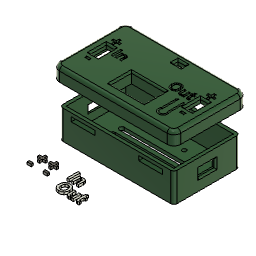
Buck Converter case v16 (Autodesk Fusion 360 design; units mm, degrees)
Autodesk Fusion 360 part; units mm, degrees
sketch "Box Main Sketch" plane through (0, 0, 0) normal (0, 0, 1) x (1, 0, 0)
  line L0 (0.0536, 74.9656) -> (0.0536, -63.0356) construction
  line L1 (-90.0982, 0.0562) -> (119.6914, 0.0562) construction
  line L2 (-33.4464, 18.5562) -> (33.5536, 18.5562)
  line L3 (33.5536, 18.5562) -> (33.5536, -18.4438)
  line L4 (33.5536, -18.4438) -> (-33.4464, -18.4438)
  line L5 (-33.4464, -18.4438) -> (-33.4464, 18.5562)
  line L6 (-35.4464, -18.4438) -> (-35.4464, 18.5562)
  line L7 (-33.4464, 20.5562) -> (33.5536, 20.5562)
  line L8 (35.5536, 18.5562) -> (35.5536, -18.4438)
  line L9 (33.5536, -20.4438) -> (-33.4464, -20.4438)
  arc A0 (35.5536, 18.5562) -> (33.5536, 20.5562) centre (33.5536, 18.5562) ccw
  arc A1 (33.5536, -20.4438) -> (35.5536, -18.4438) centre (33.5536, -18.4438) ccw
  arc A2 (-35.4464, -18.4438) -> (-33.4464, -20.4438) centre (-33.4464, -18.4438) ccw
  line L10 (-30.4464, 24.003) -> (-30.4464, 15.5562) construction
  circle A3 centre (-30.4464, 15.5562) radius 1.4
  circle A4 centre (30.5536, 15.5562) radius 1.4
  circle A5 centre (-30.4464, -15.4438) radius 1.4
  circle A6 centre (30.5536, -15.4438) radius 1.4
  line L11 (-33.4464, -18.4438) -> (-25.4464, -18.4438) construction
  line L12 (33.5536, 18.5562) -> (25.5536, 18.5562) construction
  line L13 (33.5536, 18.5562) -> (33.5536, 10.5562)
  arc A7 (-27.4464, -15.4438) -> (-25.4464, -18.4438) centre (-24.6377, -15.738) ccw
  arc A8 (-33.4464, -10.4438) -> (-30.4464, -12.4438) centre (-30.4464, -9.1938) ccw
  arc A9 (-25.4464, 18.5562) -> (-27.4464, 15.5562) centre (-24.1964, 15.5562) ccw
  arc A10 (-30.4464, 12.5562) -> (-33.4464, 10.5562) centre (-30.4464, 9.3062) ccw
  arc A11 (27.5536, 15.5562) -> (25.5536, 18.5562) centre (24.3036, 15.5562) ccw
  arc A12 (33.5536, 10.5562) -> (30.5536, 12.5562) centre (31.0441, 10.0418) ccw
  arc A13 (30.5479, -12.4438) -> (33.5536, -10.4438) centre (30.955, -9.7971) ccw
  arc A14 (25.5536, -18.4438) -> (27.5536, -15.4438) centre (24.3036, -15.4438) ccw
  arc A15 (-27.4617, -15.7469) -> (-30.4464, -12.4438) centre (-30.4464, -15.4438) ccw
  arc A16 (30.9836, -12.4748) -> (27.5536, -15.4438) centre (30.5536, -15.4438) ccw
  arc A17 (27.5536, 15.5562) -> (31.0831, 12.6033) centre (30.5536, 15.5562) ccw
  arc A18 (-30.4464, 12.5562) -> (-27.4464, 15.5562) centre (-30.4464, 15.5562) ccw
  line L14 (-20.0548, 1.2518) -> (20.324, 1.2485)
  arc A19 (20.324, 1.2485) -> (20.3242, 4.2485) centre (20.3241, 2.7485) ccw
  line L15 (20.3242, 4.2485) -> (-20.0545, 4.2518)
  arc A20 (-20.0545, 4.2518) -> (-20.0548, 1.2518) centre (-20.0547, 2.7518) ccw
  line L16 (-20.0547, -4.2975) -> (20.3241, -4.2975)
  arc A21 (20.3241, -4.2975) -> (20.3241, -1.2975) centre (20.3241, -2.7975) ccw
  line L17 (20.3241, -1.2975) -> (-20.0547, -1.2975)
  arc A22 (-20.0547, -1.2975) -> (-20.0547, -4.2975) centre (-20.0547, -2.7975) ccw
  line L18 (-20.0547, -2.7975) -> (20.3241, -2.7975) construction
  line L19 (-20.0547, 0.0562) -> (20.0734, 0.0562) construction
  line L20 (-20.0547, -9.6836) -> (20.3241, -9.6836)
  arc A23 (20.3241, -9.6836) -> (20.3241, -6.6836) centre (20.3241, -8.1836) ccw
  line L21 (20.3241, -6.6836) -> (-20.0547, -6.6836)
  arc A24 (-20.0547, -6.6836) -> (-20.0547, -9.6836) centre (-20.0547, -8.1836) ccw
  line L22 (-20.0547, -8.1836) -> (20.3241, -8.1836) construction
  line L23 (-20.0547, -15.4896) -> (20.3241, -15.4896)
  arc A25 (20.3241, -15.4896) -> (20.3241, -12.4896) centre (20.3241, -13.9896) ccw
  line L24 (20.3241, -12.4896) -> (-20.0547, -12.4896)
  arc A26 (-20.0547, -12.4896) -> (-20.0547, -15.4896) centre (-20.0547, -13.9896) ccw
  line L25 (-20.0547, -13.9896) -> (20.3241, -13.9896) construction
  arc A27 (-33.4464, 20.5562) -> (-35.4464, 18.5562) centre (-33.4464, 18.5562) ccw
  line L26 (-33.4464, 5.5562) -> (-35.4464, 5.5562)
  line L27 (35.5536, 5.5562) -> (33.5536, 5.5562)
  line L28 (35.5536, 7.5562) -> (33.5536, 7.5562) construction
  line L29 (-33.4464, 7.5562) -> (-35.4464, 7.5562) construction
  circle A28 centre (-29.0547, 10.5065) radius 1.25
  line L30 (-29.0547, 10.5065) -> (22.3046, 10.5554) construction
  line L31 (-14.904, 20.5562) -> (-14.904, 11.5562) construction
  circle A29 centre (11.0453, 10.5447) radius 1.25
  line L32 (-29.0547, 10.5065) -> (-29.0547, 26.528) construction
  line L33 (11.0453, 10.5447) -> (11.0453, 25.7111) construction
  line L34 (-29.0547, 24.003) -> (11.0453, 24.003) construction
  point P0 (30.5536, -15.4438)
  dimension "d1" = 67
  dimension "d2" = 37
  dimension "d4" = 2
  dimension "d9" = 2.8
  dimension "d65" = 3
  dimension "d66" = 3
  dimension "d68" = 3
  dimension "d69" = 3
  dimension "d80" = 2
  dimension "d82" = 2
  dimension "d83" = 2
  dimension "d181" = 2.5
  dimension "d194" = 9
  dimension "d195" = 2.5
  dimension "d206" = 40.1
  constraint vertical L0
  constraint perpendicular L0 L1
  constraint horizontal L2
  constraint vertical L3
  constraint horizontal L4
  constraint vertical L5
  constraint symmetric L0 L3 L5
  constraint symmetric L1 L2 L4
  constraint tangent L7 A0
  constraint tangent L8 A0
  constraint tangent L8 A1
  constraint tangent L9 A1
  constraint equal A0 A1
  constraint tangent L6 A2
  constraint tangent L9 A2
  constraint equal A0 A2
  constraint coincident L10.end A3.centre
  constraint coincident L4.end L5.start
  constraint coincident L4 L11.end
  constraint coincident L2.end L3.start
  constraint perpendicular L2 L13
  constraint coincident A7.start A15
  constraint tangent A8 A15
  constraint coincident L5 A8.start
  constraint tangent A9 A18
  constraint coincident L2 A9.start
  constraint tangent A10 A18
  constraint coincident L5 A10.end
  constraint tangent A11 A17
  constraint coincident A12.end A17
  constraint coincident L3 A13.end
  constraint coincident A13.start A16
  constraint tangent A14 A16
  constraint coincident L4 A14.start
  constraint coincident A7 A15.start
  constraint concentric A6 A16
  constraint coincident A13 A16.start
  constraint coincident A12 A17.end
  constraint tangent L14 A19
  constraint tangent A19 L15
  constraint parallel L14 L15
  constraint tangent L15 A20
  constraint tangent L14 A20
  constraint tangent L16 A21
  constraint tangent A21 L17
  constraint parallel L16 L17
  constraint tangent L17 A22
  constraint tangent L16 A22
  constraint coincident L1 L19.start
  constraint tangent L20 A23
  constraint tangent A23 L21
  constraint parallel L20 L21
  constraint tangent L21 A24
  constraint tangent L20 A24
  constraint tangent L23 A25
  constraint tangent A25 L24
  constraint parallel L23 L24
  constraint tangent L24 A26
  constraint tangent L23 A26
  constraint tangent L6 A27
  constraint tangent L7 A27
  constraint coincident L5 L26.start
  constraint coincident L6 L26.end
  constraint perpendicular L6 L26
  constraint coincident L8 L27.start
  constraint coincident L3 L27.end
  constraint coincident L7 L31.start
  constraint perpendicular L2 L31
  constraint coincident L30 A29.centre
  constraint coincident A28.centre L30.start
  constraint perpendicular L2 L32
  constraint coincident A29.centre L33.start
  constraint perpendicular L7 L33
  constraint coincident L32 L34.start
  constraint coincident L33 L34.end
  constraint perpendicular L33 L34
  measures "d1" distance of L2.start L2.end
  measures "d2" distance of L2.start L4.end
  measures "d4" radius of A0
  measures "d9" diameter of A3
  measures "d65" diameter of A19
  measures "d66" diameter of A21
  measures "d68" diameter of A23
  measures "d69" diameter of A25
  measures "d80" radius of A27
  measures "d82" distance of L27
  measures "d83" distance of L26
  measures "d181" diameter of A28
  measures "d194" distance of L31.start L31.end
  measures "d195" diameter of A29
  measures "d206" distance of L34.start L34.end
extrude "Bottom of Box" add sketch "Box Main Sketch" along normal blind 2 contours L2 L3 L4 L5 A7 A8 A9 A10 A11 A12 A13 A14 A15 A16 A17 A18 | L14 A19 L15 A20 | L16 A21 L17 A22 | L20 A23 L21 A24 | L23 A25 L24 A26 | A28 | A29 makes body 1
extrude "Bottom Corners" add sketch "Box Main Sketch" along normal blind 5 contours L2 L5 A9 A10 A18 | L2 L3 L13 A11 A12 A17 | L4 L5 A7 A8 A15 | L3 L4 A13 A14 A16 | A3 | A4 | A5 | A6 bodies 1
extrude "Main Box Body" add sketch "Box Main Sketch" along normal blind 18 contours L2 L3 L5 L6 L7 L8 A0 L13 A27 L26 L27 | L3 L4 L5 L6 L8 L9 A1 A2 L26 L27 bodies 1
sketch "End of Box for input" plane through (33.5536, 0, 0) normal (-1, 0, 0) x (0, -1, 0)
  line L0 (10.4438, 5) -> (18.4438, 5)
  line L1 (18.4438, 5) -> (18.4438, 18)
  line L2 (18.4438, 18) -> (-18.5562, 18)
  line L3 (-18.5562, 18) -> (-18.5562, 5)
  line L4 (-18.5562, 5) -> (-10.5562, 5)
  line L5 (-10.5562, 5) -> (-10.5562, 2)
  line L6 (-10.5562, 2) -> (10.4438, 2)
  line L7 (10.4438, 2) -> (10.4438, 5)
  line L8 (4.6555, 6.9963) -> (-5.3445, 6.9963)
  line L9 (-5.3445, 6.9963) -> (-5.3445, 11.9963)
  line L10 (-5.3445, 11.9963) -> (4.6555, 11.9963)
  line L11 (4.6555, 11.9963) -> (4.6555, 6.9963)
  line L12 (0, 0) -> (0, 7) construction
  dimension "d54" = 10
  dimension "d55" = 5
  dimension "d72" = 7
  constraint horizontal L8
  constraint vertical L9
  constraint horizontal L10
  constraint vertical L11
  constraint coincident L12.start origin
  constraint perpendicular L0 L12
  measures "d54" distance of L8.start L8.end
  measures "d55" distance of L8.start L10.end
  measures "d72" distance of L12.start L12.end
extrude "End Wire Holes" cut sketch "End of Box for input" against normal blind 2 contours L8 L9 L10 L11 bodies 1
sketch "End of box for output" plane through (-35.4464, 0, 0) normal (-1, 0, 0) x (0, -1, 0)
  line L0 (-18.5562, 0) -> (18.4438, 0)
  line L1 (18.4438, 0) -> (18.4438, 18)
  line L2 (18.4438, 18) -> (-18.5562, 18)
  line L3 (-5.1039, 6.9396) -> (4.8961, 6.9396)
  line L4 (4.8961, 6.9396) -> (4.8961, 11.9396)
  line L5 (4.8961, 11.9396) -> (-5.1039, 11.9396)
  line L6 (-5.1039, 11.9396) -> (-5.1039, 6.9396)
  line L7 (3.7468, 0) -> (3.7468, 7) construction
  line L8 (-18.5562, 18) -> (-18.5562, 0)
  dimension "d43" = 10
  dimension "d44" = 5
  dimension "d58" = 7
  constraint horizontal L3
  constraint vertical L4
  constraint horizontal L5
  constraint vertical L6
  constraint coincident L0 L7.start
  constraint perpendicular L3 L7
  measures "d43" distance of L3.start L3.end
  measures "d44" distance of L3.start L5.end
  measures "d58" distance of L7.start L7.end
extrude "End Wire Hole" cut sketch "End of box for output" against normal blind 2 contours L3 L4 L5 L6 bodies 1
fillet "wire Hole" radius 1 4 edges at (-35.4464, 0.1039, 11.9396) (-35.4464, 5.1039, 9.4396) (-35.4464, 0.1039, 6.9396) (-35.4464, -4.8961, 9.4396) on bodies 1
fillet "Wire Hole" radius 1 4 edges at (35.5536, 0.3445, 6.9963) (35.5536, 5.3445, 9.4963) (35.5536, 0.3445, 11.9963) (35.5536, -4.6555, 9.4963) on bodies 1
extrude "Mounting Posts" add sketch "Box Main Sketch" along normal blind 8 contours A3 | A4 | A5 | A6 bodies 1
extrude "Vent Holes in bottom" cut sketch "Box Main Sketch" along normal blind 2 contours L14 A19 L15 A20 | L16 A21 L17 A22 | L20 A23 L21 A24 | L23 A25 L24 A26 bodies 1
sketch "Box Catch holes" plane through (0, 20.5562, 0) normal (0, 1, 0) x (-1, 0, 0)
  line L0 (-33.5536, 0) -> (33.4464, 0)
  line L1 (33.4464, 0) -> (33.4464, 18)
  line L2 (33.4464, 18) -> (-33.5536, 18)
  line L3 (-33.5536, 18) -> (-33.5536, 0)
  line L4 (33.4464, 16.015) -> (28.4464, 16.015) construction
  line L5 (28.4464, 16.015) -> (13.4464, 16.015)
  line L6 (13.4464, 16.015) -> (13.4464, 13.015)
  line L7 (13.4464, 13.015) -> (28.4464, 13.015)
  line L8 (28.4464, 13.015) -> (28.4464, 16.015)
  line L9 (-28.5536, 13.0366) -> (-13.5536, 13.0366)
  line L10 (-28.5536, 16.0366) -> (-28.5536, 13.0366)
  line L11 (-13.5536, 16.0366) -> (-28.5536, 16.0366)
  line L12 (-13.5536, 13.0366) -> (-13.5536, 16.0366)
  dimension "d85" = 5
  dimension "d87" = 15
  dimension "d88" = 3
  dimension "d89" = 15
  dimension "d90" = 3
  constraint coincident L1 L4.start
  constraint perpendicular L1 L4
  constraint horizontal L5
  constraint vertical L6
  constraint horizontal L7
  constraint vertical L8
  constraint horizontal L11
  constraint vertical L10
  constraint horizontal L9
  constraint vertical L12
  measures "d85" distance of L4.start L4.end
  measures "d87" distance of L4.end L5.end
  measures "d88" distance of L4.end L7.end
  measures "d89" distance of L10.start L11.start
  measures "d90" distance of L9.end L11.start
extrude "Back Catch Slots" cut sketch "Box Catch holes" against normal blind 1.5 draft -45 contours L5 L6 L7 L8 | L9 L10 L11 L12 bodies 1
mirror "Front Catches" about plane through (0, 0, 0) normal (0, 1, 0) of "Back Catch Slots"
sketch "Lid Rim" plane through (0, 0, 18) normal (0, 0, 1) x (-1, 0, 0) in component "Lid"
  line L0 (33.4464, -18.5562) -> (-33.5536, -18.5562)
  line L1 (-33.5536, -18.5562) -> (-33.5536, 18.4438)
  line L2 (-33.5536, 18.4438) -> (33.4464, 18.4438)
  line L3 (33.4464, 18.4438) -> (33.4464, -18.5562)
  arc A0 (-35.5536, -18.5562) -> (-33.5536, -20.5562) centre (-33.5536, -18.5562) ccw
  line L4 (-33.5536, -20.5562) -> (33.4464, -20.5562)
  arc A1 (33.4464, -20.5562) -> (35.4464, -18.5562) centre (33.4464, -18.5562) ccw
  line L5 (35.4464, -18.5562) -> (35.4464, 18.4438)
  arc A2 (35.4464, 18.4438) -> (33.4464, 20.4438) centre (33.4464, 18.4438) ccw
  line L6 (33.4464, 20.4438) -> (-33.5536, 20.4438)
  arc A3 (-33.5536, 20.4438) -> (-35.5536, 18.4438) centre (-33.5536, 18.4438) ccw
  line L7 (-35.5536, 18.4438) -> (-35.5536, -18.5562)
  line L8 (-33.5536, 20.4438) -> (33.4464, 20.4438)
  arc A4 (-33.5536, 20.4438) -> (-35.5536, 18.4438) centre (-33.5536, 18.4438) ccw
  line L9 (-35.5536, -18.5562) -> (-35.5536, 18.4438)
  arc A5 (-35.5536, -18.5562) -> (-33.5536, -20.5562) centre (-33.5536, -18.5562) ccw
  line L10 (33.4464, -20.5562) -> (-33.5536, -20.5562)
  arc A6 (33.4464, -20.5562) -> (35.4464, -18.5562) centre (33.4464, -18.5562) ccw
  line L11 (35.4464, 18.4438) -> (35.4464, -18.5562)
  arc A7 (35.4464, 18.4438) -> (33.4464, 20.4438) centre (33.4464, 18.4438) ccw
  line L12 (-37.7536, 18.4438) -> (-37.7536, -18.5562)
  arc A8 (-37.7536, -18.5562) -> (-33.5536, -22.7562) centre (-33.5536, -18.5562) ccw
  line L13 (-33.5536, -22.7562) -> (33.4464, -22.7562)
  arc A9 (33.4464, -22.7562) -> (37.6464, -18.5562) centre (33.4464, -18.5562) ccw
  line L14 (37.6464, -18.5562) -> (37.6464, 18.4438)
  arc A10 (37.6464, 18.4438) -> (33.4464, 22.6438) centre (33.4464, 18.4438) ccw
  line L15 (33.4464, 22.6438) -> (-33.5536, 22.6438)
  arc A11 (-33.5536, 22.6438) -> (-37.7536, 18.4438) centre (-33.5536, 18.4438) ccw
  line L16 (-35.7536, 18.4438) -> (-35.7536, -18.5562)
  arc A12 (-35.7536, -18.5562) -> (-33.5536, -20.7562) centre (-33.5536, -18.5562) ccw
  line L17 (-33.5536, -20.7562) -> (33.4464, -20.7562)
  arc A13 (33.4464, -20.7562) -> (35.6464, -18.5562) centre (33.4464, -18.5562) ccw
  line L18 (35.6464, -18.5562) -> (35.6464, 18.4438)
  arc A14 (35.6464, 18.4438) -> (33.4464, 20.6438) centre (33.4464, 18.4438) ccw
  line L19 (33.4464, 20.6438) -> (-33.5536, 20.6438)
  arc A15 (-33.5536, 20.6438) -> (-35.7536, 18.4438) centre (-33.5536, 18.4438) ccw
  constraint concentric A0 A8
  constraint concentric A1 A9
  constraint concentric A2 A10
  constraint concentric A3 A11
  constraint tangent L15 A11
  constraint tangent L14 A10
  constraint tangent A9 L14
  constraint tangent L13 A9
  constraint tangent A8 L13
  constraint tangent A10 L15
  constraint tangent L12 A8
  constraint tangent L12 A11
  constraint concentric A0 A12
  constraint concentric A1 A13
  constraint concentric A2 A14
  constraint concentric A3 A15
  constraint tangent A14 L19
  constraint tangent L18 A14
  constraint tangent L19 A15
  constraint tangent A13 L18
  constraint tangent L16 A15
  constraint tangent L17 A13
  constraint tangent A12 L17
  constraint tangent L16 A12
extrude "Lid Main Part" add sketch "Lid Rim" against normal blind 5 separate body contours L12 A8 L13 A9 L14 A10 L15 A11 makes body 2 in component "Lid"
sketch "Lid top" plane through (0, 0, 18) normal (0, 0, 1) x (1, 0, 0) in component "Lid"
  line L0 (33.5536, 22.7562) -> (-33.4464, 22.7562)
  arc A0 (37.7536, 18.5562) -> (33.5536, 22.7562) centre (33.5536, 18.5562) ccw
  line L1 (37.7536, -18.4438) -> (37.7536, 18.5562)
  arc A1 (33.5536, -22.6438) -> (37.7536, -18.4438) centre (33.5536, -18.4438) ccw
  line L2 (-33.4464, -22.6438) -> (33.5536, -22.6438)
  arc A2 (-37.6464, -18.4438) -> (-33.4464, -22.6438) centre (-33.4464, -18.4438) ccw
  line L3 (-37.6464, 18.5562) -> (-37.6464, -18.4438)
  arc A3 (-33.4464, 22.7562) -> (-37.6464, 18.5562) centre (-33.4464, 18.5562) ccw
  line L4 (31.7125, -5.0985) -> (26.7125, -5.0985)
  line L5 (26.7125, -5.0985) -> (26.7125, 4.9015)
  line L6 (26.7125, 4.9015) -> (31.7125, 4.9015)
  line L7 (31.7125, 4.9015) -> (31.7125, -5.0985)
  line L8 (-37.6464, 2.2618) -> (-33.6464, 2.2618) construction
  line L9 (-26.7875, 4.9015) -> (-26.7875, -5.0985)
  line L10 (-26.7875, -5.0985) -> (-31.7875, -5.0985)
  line L11 (-31.7875, -5.0985) -> (-31.7875, 4.9015)
  line L12 (-31.7875, 4.9015) -> (-26.7875, 4.9015)
  line L13 (-0.6158, 18.2562) -> (4.3842, 18.2562)
  line L14 (4.3842, 18.2562) -> (4.3842, 15.2562)
  line L15 (4.3842, 15.2562) -> (-0.6158, 15.2562)
  line L16 (-0.6158, 15.2562) -> (-0.6158, 18.2562)
  line L17 (-35.4464, 18.5562) -> (-35.4464, -18.4438)
  line L18 (33.5536, 20.5562) -> (-33.4464, 20.5562)
  line L19 (35.5536, -18.4438) -> (35.5536, 18.5562)
  line L20 (-33.4464, -20.4438) -> (33.5536, -20.4438)
  line L21 (-35.4464, -18.4438) -> (-35.4464, 18.5562)
  line L22 (-33.4464, 20.5562) -> (33.5536, 20.5562)
  line L23 (33.5536, -20.4438) -> (-33.4464, -20.4438)
  line L24 (35.5536, 18.5562) -> (35.5536, -18.4438)
  line L25 (-8.8611, -20.4438) -> (-8.8611, -15.4438) construction
  line L26 (-8.8611, -15.4438) -> (12.1389, -15.4438)
  line L27 (12.1389, -15.4438) -> (12.1389, -2.4438)
  line L28 (12.1389, -2.4438) -> (-8.8611, -2.4438)
  line L29 (-8.8611, -2.4438) -> (-8.8611, -15.4438)
  line L30 (-10.3611, -0.9438) -> (-10.3611, -16.9438)
  line L31 (-10.3611, -16.9438) -> (13.6389, -16.9438)
  line L32 (13.6389, -16.9438) -> (13.6389, -0.9438)
  line L33 (13.6389, -0.9438) -> (-10.3611, -0.9438)
  line L34 (22.4453, -20.4438) -> (22.4453, -13.9438) construction
  line L35 (24.0234, -12.7383) -> (24.0234, -2.5519)
  line L36 (24.0234, -2.5519) -> (20.8495, -2.5519)
  line L37 (20.8495, -2.5519) -> (20.8495, -12.7383)
  line L38 (25.0234, -12.4097) -> (25.0234, -3.5519)
  line L39 (19.8495, -3.5519) -> (19.8495, -12.4399)
  arc A4 (19.8495, -12.4399) -> (25.0234, -12.4097) centre (22.4453, -13.9438) ccw
  arc A5 (20.8495, -12.7383) -> (24.0234, -12.7152) centre (22.4453, -13.9438) ccw
  line L40 (20.8495, -2.5519) -> (19.7948, -3.6066)
  line L41 (20.8495, -2.5519) -> (22.3411, -2.5519) construction
  line L42 (24.0234, -2.5519) -> (24.9601, -3.4885)
  line L43 (25.0234, -2.5519) -> (25.348, -2.5519) construction
  line L44 (24.9601, -3.4885) -> (25.0234, -3.5519)
  circle A6 centre (22.4453, -13.9438) radius 1.875
  dimension "d113" = 5
  dimension "d114" = 10
  dimension "d116" = 4
  dimension "d117" = 5
  dimension "d118" = 10
  dimension "d121" = 5
  dimension "d122" = 3
  dimension "d126" = 5
  dimension "d127" = 21
  dimension "d128" = 13
  dimension "d129" = 1.5
  dimension "d143" = 6.5
  dimension "d144" = 4
  dimension "d147" = 135
  dimension "d148" = 45
  dimension "d149" = 3.75
  constraint horizontal L4
  constraint vertical L5
  constraint horizontal L6
  constraint vertical L7
  constraint coincident L3 L8.start
  constraint perpendicular L3 L8
  constraint horizontal L10
  constraint vertical L11
  constraint horizontal L12
  constraint vertical L9
  constraint horizontal L13
  constraint vertical L14
  constraint horizontal L15
  constraint vertical L16
  constraint coincident L20 L25.start
  constraint perpendicular L20 L25
  constraint horizontal L26
  constraint vertical L27
  constraint horizontal L28
  constraint vertical L29
  constraint coincident L23 L34.start
  constraint perpendicular L23 L34
  constraint coincident L34.end A4.centre
  constraint vertical L35
  constraint horizontal L36
  constraint vertical L37
  constraint concentric A4 A5
  constraint coincident L35 A5.end
  constraint horizontal L41
  constraint coincident L40 L39.start
  constraint horizontal L43
  constraint parallel L42 L44
  constraint concentric A4 A6
  measures "d113" distance of L4.start L4.end
  measures "d114" distance of L4.start L6.end
  measures "d116" distance of L8.start L8.end
  measures "d117" distance of L9.end L10.end
  measures "d118" distance of L9.end L9.start
  measures "d121" distance of L13.start L13.end
  measures "d122" distance of L13.start L15.end
  measures "d126" distance of L25.start L25.end
  measures "d127" distance of L25.end L26.end
  measures "d128" distance of L25.end L28.end
  measures "d143" distance of L34.start L34.end
  measures "d144" diameter of A5
  measures "d147" angle of L40 L41
  measures "d148" angle of L42 L43
  measures "d149" diameter of A6
extrude "Lid top (1)" add sketch "Lid top" along normal blind 3 contours L0 A0 L1 A1 L2 A2 L3 A3 | L4 L5 L6 L7 | L9 L10 L11 L12 | L13 L14 L15 L16 | L26 L27 L28 L29 | L30 L31 L32 L33 | L35 L36 L37 A5 | L35 L37 L38 L39 A4 A5 L40 L42 L44 | A6 bodies 2 in component "Lid"
fillet "Lid top (2)" radius 2 1 faces at (11.2203, -7.5105, 21) on bodies 2 in component "Lid"
sketch "Lid Catches" plane through (0, -20.6438, 0) normal (0, 1, 0) x (-1, 0, 0) in component "Lid"
  line L0 (33.4464, 18) -> (-33.5536, 18)
  line L1 (-33.5536, 18) -> (-33.5536, 13)
  line L2 (-33.5536, 13) -> (33.4464, 13)
  line L3 (33.4464, 13) -> (33.4464, 18)
  line L4 (-13.5536, 16.0366) -> (-13.5536, 13.0366)
  line L5 (-13.5536, 13.0366) -> (-28.5536, 13.0366)
  line L6 (-28.5536, 13.0366) -> (-28.5536, 16.0366)
  line L7 (13.4464, 13.015) -> (13.4464, 16.015)
  line L8 (28.4464, 13.015) -> (13.4464, 13.015)
  line L9 (28.4464, 16.015) -> (28.4464, 13.015)
  line L10 (-13.5536, 16.0366) -> (-28.5536, 16.0366)
  line L11 (-13.5536, 13.0366) -> (-13.5536, 16.0366)
  line L12 (-28.5536, 13.0366) -> (-13.5536, 13.0366)
  line L13 (-28.5536, 16.0366) -> (-28.5536, 13.0366)
  line L14 (13.4464, 16.015) -> (13.4464, 13.015)
  line L15 (13.4464, 13.015) -> (28.4464, 13.015)
  line L16 (28.4464, 13.015) -> (28.4464, 16.015)
  line L17 (28.4464, 16.015) -> (13.4464, 16.015)
extrude "Front Catch Pins" add sketch "Lid Catches" along normal blind 1.5 draft -45 contours L4 L5 L6 L10 L11 L12 L13 | L7 L8 L9 L14 L15 L16 L17 bodies 2 in component "Lid"
sketch "Other Lid Catches" plane through (0, 20.7562, 0) normal (0, -1, 0) x (1, 0, 0) in component "Lid"
  line L0 (33.5536, 18) -> (-33.4464, 18)
  line L1 (-33.4464, 18) -> (-33.4464, 13)
  line L2 (-33.4464, 13) -> (33.5536, 13)
  line L3 (33.5536, 13) -> (33.5536, 18)
  line L4 (28.4413, 15.9243) -> (28.4413, 13.149)
  line L5 (13.666, 15.9243) -> (28.4413, 15.9243)
  line L6 (13.666, 13.149) -> (13.666, 15.9243)
  line L7 (13.666, 15.9243) -> (28.4413, 15.9243)
  line L8 (28.4413, 15.9243) -> (28.4413, 13.149)
  line L9 (28.4413, 13.149) -> (13.666, 13.149)
  line L10 (13.666, 13.149) -> (13.666, 15.9243)
  line L11 (-28.334, 15.9026) -> (-13.5587, 15.9026)
  line L12 (-13.5587, 15.9026) -> (-13.5587, 13.1274)
  line L13 (-13.5587, 13.1274) -> (-28.334, 13.1274)
  line L14 (-28.334, 13.1274) -> (-28.334, 15.9026)
  line L15 (-33.4464, 0) -> (33.5536, 0)
  line L16 (33.5536, 0) -> (33.5536, 18)
  line L17 (33.5536, 18) -> (-33.4464, 18)
  line L18 (-33.4464, 18) -> (-33.4464, 0)
  line L19 (-13.5587, 15.9026) -> (-13.5587, 13.1274)
  line L20 (-28.334, 15.9026) -> (-13.5587, 15.9026)
  line L21 (-28.334, 13.1274) -> (-28.334, 15.9026)
  line L22 (-13.5587, 13.1274) -> (-28.334, 13.1274)
extrude "Rear Catch Pins" add sketch "Other Lid Catches" along normal blind 1.5 draft -45 contours L4 L5 L6 L7 L8 L9 L10 | L11 L12 L13 L14 L19 L20 L21 L22 bodies 2 in component "Lid"
extrude "Top Holes" cut sketch "Lid top" along normal blind 3 contours L4 L5 L6 L7 | L9 L10 L11 L12 | L13 L14 L15 L16 | L26 L27 L28 L29 | L35 L37 L38 L39 A4 A5 L40 L42 L44 bodies 2 in component "Lid"
extrude "Voltage Display hole" add sketch "Lid top" against normal blind 3.7 contours L30 L31 L32 L33 bodies 2 in component "Lid"
fillet "Screw Holes" radius 1 15 edges at (-26.7875, -0.0985, 21) (-29.2875, 4.9015, 21) (-31.7875, -0.0985, 21) (-29.2875, -5.0985, 21) (1.6389, -2.4438, 21) (-8.8611, -8.9438, 21) (1.6389, -15.4438, 21) (1.8842, 15.2562, 21) (26.7125, -0.0985, 21) (29.2125, -5.0985, 21) (31.7125, -0.0985, 21) (29.2125, 4.9015, 21) (4.3842, 16.7562, 21) (1.8842, 18.2562, 21) (-0.6158, 16.7562, 21) on bodies 2 in component "Lid"
fillet "Voltage Display" radius 1 1 edges at (12.1389, -8.9438, 21) on bodies 2 in component "Lid"
move_body "Move1" bodies 2 to x (1, 0, 0) y (0, 1, 0) z (0, 0, 1) at (0, 0, 35) in component "Lid"
move_body "Move2" bodies 2 to x (1, 0, 0) y (0, 1, 0) z (0, 0, 1) at (0, 0, -35) in component "Lid"
extrude "PushButton Pin" add sketch "Lid top" against normal blind 5.75 draft -3 contours A6 bodies 2 in component "Lid"
sketch "Emboss Letters" plane through (0, 0, 21) normal (0, 0, 1) x (-1, 0, 0) in component "Lid"
  arc A0 (33.4464, -20.7562) -> (35.6464, -18.5562) centre (33.4464, -18.5562) ccw
  line L0 (35.6464, -18.5562) -> (35.6464, 18.4438)
  arc A1 (35.6464, 18.4438) -> (33.4464, 20.6438) centre (33.4464, 18.4438) ccw
  line L1 (33.4464, 20.6438) -> (-33.5536, 20.6438)
  arc A2 (-33.5536, 20.6438) -> (-35.7536, 18.4438) centre (-33.5536, 18.4438) ccw
  line L2 (-35.7536, 18.4438) -> (-35.7536, -18.5562)
  arc A3 (-35.7536, -18.5562) -> (-33.5536, -20.7562) centre (-33.5536, -18.5562) ccw
  line L3 (-33.5536, -20.7562) -> (33.4464, -20.7562)
  line L4 (31.8884, -5.9664) -> (26.4793, -6.0573) construction
  line L5 (26.4793, -6.0573) -> (26.568, -11.3367) construction
  line L6 (26.568, -11.3367) -> (31.9771, -11.2458) construction
  line L7 (31.9771, -11.2458) -> (31.8884, -5.9664) construction
  line L8 (-27.1116, -5.9664) -> (-32.5207, -6.0573) construction
  line L9 (-32.5207, -6.0573) -> (-32.432, -11.3367) construction
  line L10 (-32.432, -11.3367) -> (-27.0229, -11.2458) construction
  line L11 (-27.0229, -11.2458) -> (-27.1116, -5.9664) construction
  line L12 (24.0133, 0.021) -> (14.3092, 0.0016) construction
  line L13 (14.3092, 0.0016) -> (14.3216, -6.2061) construction
  line L14 (14.3216, -6.2061) -> (24.0257, -6.1867) construction
  line L15 (24.0257, -6.1867) -> (24.0133, 0.021) construction
  line L16 (-10.495, 0.0928) -> (-24.7584, 0.1552) construction
  line L17 (-24.7584, 0.1552) -> (-24.7855, -6.0483) construction
  line L18 (-24.7855, -6.0483) -> (-10.5221, -6.1106) construction
  line L19 (-10.5221, -6.1106) -> (-10.495, 0.0928) construction
  line L20 (-13.1389, 16.4438) -> (9.8611, 16.4438)
  line L21 (9.8611, 16.4438) -> (9.8611, 1.4438)
  line L22 (9.8611, 1.4438) -> (-13.1389, 1.4438)
  line L23 (-13.1389, 1.4438) -> (-13.1389, 16.4438)
  line L24 (-5.3842, -19.2562) -> (-5.3842, -14.2562)
  line L25 (-5.3842, -14.2562) -> (1.6158, -14.2562)
  line L26 (1.6158, -14.2562) -> (1.6158, -19.2562)
  line L27 (1.6158, -19.2562) -> (-5.3842, -19.2562)
  line L28 (32.7875, -5.9015) -> (25.7875, -5.9015)
  line L29 (25.7875, -5.9015) -> (25.7875, 6.0985)
  line L30 (25.7875, 6.0985) -> (32.7875, 6.0985)
  line L31 (32.7875, 6.0985) -> (32.7875, -5.9015)
  line L32 (-20.8495, 2.5519) -> (-20.8495, 12.7383)
  arc A4 (-20.8495, 12.7383) -> (-24.0234, 12.7152) centre (-22.4453, 13.9438) ccw
  line L33 (-24.0234, 12.7152) -> (-24.0234, 2.5519)
  line L34 (-24.0234, 2.5519) -> (-25.0234, 3.5519)
  line L35 (-25.0234, 3.5519) -> (-25.0234, 12.4097)
  arc A5 (-19.8495, 12.4399) -> (-25.0234, 12.4097) centre (-22.4453, 13.9438) ccw
  line L36 (-19.8495, 12.4399) -> (-19.8495, 3.5519)
  line L37 (-19.8495, 3.5519) -> (-20.8495, 2.5519)
  line L38 (-32.7125, -5.9015) -> (-32.7125, 6.0985)
  line L39 (-32.7125, 6.0985) -> (-25.7125, 6.0985)
  line L40 (-25.7125, 6.0985) -> (-25.7125, -5.9015)
  line L41 (-25.7125, -5.9015) -> (-32.7125, -5.9015)
  line L42 (31.0051, 10.7007) -> (25.4979, 10.7007) construction
  line L43 (25.4979, 10.7007) -> (25.4979, 8.0454) construction
  line L44 (25.4979, 8.0454) -> (31.0051, 8.0454) construction
  line L45 (31.0051, 8.0454) -> (31.0051, 10.7007) construction
  line L46 (-27.9949, 10.7007) -> (-33.5021, 10.7007) construction
  line L47 (-33.5021, 10.7007) -> (-33.5021, 8.0454) construction
  line L48 (-33.5021, 8.0454) -> (-27.9949, 8.0454) construction
  line L49 (-27.9949, 8.0454) -> (-27.9949, 10.7007) construction
  dimension "d170" = 7
  dimension "d172" = 7
  dimension "d175" = 6
  dimension "d176" = 6
  dimension "d188" = 7
  dimension "d189" = 7
  text T0 "+" font "Arial" height 7 bold align left top in box 5.4099 x 5.2802 at (31.8884, -5.9664) x (-0.999859, -0.016798) y (0.016798, -0.999859) spacing 1 kerned
  text T1 "+" font "Arial" height 7 bold align left top in box 5.4099 x 5.2802 at (-27.1116, -5.9664) x (-0.999859, -0.016798) y (0.016798, -0.999859) spacing 1 kerned
  text T2 "In" font "Arial" height 6 bold align left top in box 9.7041 x 6.2077 at (24.0133, 0.021) x (-0.999998, -0.001996) y (0.001996, -0.999998) spacing 1 kerned
  text T3 "Out" font "Arial" height 6 bold align left top in box 14.2635 x 6.2035 at (-10.495, 0.0928) x (-0.99999, 0.004371) y (-0.004371, -0.99999) spacing 1 kerned
  text T4 "-" font "Arial" height 7 bold align left top in box 5.5072 x 2.6552 at (31.0051, 10.7007) x (-1, 0) y (0, -1) spacing 1 kerned
  text T5 "-" font "Arial" height 7 bold align left top in box 5.5072 x 2.6552 at (-27.9949, 10.7007) x (-1, 0) y (0, -1) spacing 1 kerned
move_body "Move3" bodies 2 to x (1, 0, 0) y (0, 1, 0) z (0, 0, 1) at (0, 0, 24) in component "Lid"
move_body "Move4" bodies 2 to x (1, 0, 0) y (0, 1, 0) z (0, 0, 1) at (0, 0, -25) in component "Lid"
move_body "Move5" bodies 2 to x (1, 0, 0) y (0, 1, 0) z (0, 0, 1) at (0, 0, 1) in component "Lid"
extrude "Bottom Mounting Holes" cut sketch "Box Main Sketch" along normal blind 2 contours A28 bodies 1
emboss "Emboss3" depth -1.5 profiles "Emboss Letters" section 1 text T0 T4 T2 T3 T5 T1 onto face at (-20.2832, 15.3046, 21) on bodies 2 bodies 2 in component "Lid"
extrude "Mounting Holes" cut sketch "Box Main Sketch" along normal blind 2 contours A29 bodies 1
sketch "text Fills" plane through (0, 0, 0) normal (0, 0, 1) x (1, 0, 0)
  line L0 (-31.9332, -38.7504) -> (-26.4316, -38.7504) construction
  line L1 (-26.4316, -38.7504) -> (-26.4316, -34.684) construction
  line L2 (-26.4316, -34.684) -> (-31.9332, -34.684) construction
  line L3 (-31.9332, -34.684) -> (-31.9332, -38.7504) construction
  line L4 (-24.9332, -38.7504) -> (-19.4316, -38.7504) construction
  line L5 (-19.4316, -38.7504) -> (-19.4316, -34.684) construction
  line L6 (-19.4316, -34.684) -> (-24.9332, -34.684) construction
  line L7 (-24.9332, -34.684) -> (-24.9332, -38.7504) construction
  line L8 (-32.1724, -45.0892) -> (-25.4748, -45.0892) construction
  line L9 (-25.4748, -45.0892) -> (-25.4748, -42.6972) construction
  line L10 (-25.4748, -42.6972) -> (-32.1724, -42.6972) construction
  line L11 (-32.1724, -42.6972) -> (-32.1724, -45.0892) construction
  line L12 (-22.1724, -45.0892) -> (-15.4748, -45.0892) construction
  line L13 (-15.4748, -45.0892) -> (-15.4748, -42.6972) construction
  line L14 (-15.4748, -42.6972) -> (-22.1724, -42.6972) construction
  line L15 (-22.1724, -42.6972) -> (-22.1724, -45.0892) construction
  line L16 (-11.0032, -40.066) -> (1.3156, -40.066) construction
  line L17 (1.3156, -40.066) -> (1.3156, -33.488) construction
  line L18 (1.3156, -33.488) -> (-11.0032, -33.488) construction
  line L19 (-11.0032, -33.488) -> (-11.0032, -40.066) construction
  line L20 (-10.166, -47.9597) -> (3.4684, -47.9597) construction
  line L21 (3.4684, -47.9597) -> (3.4684, -42.6972) construction
  line L22 (3.4684, -42.6972) -> (-10.166, -42.6972) construction
  line L23 (-10.166, -42.6972) -> (-10.166, -47.9597) construction
  dimension "d198" = 6.9
  dimension "d199" = 6.9
  dimension "d200" = 6.9
  dimension "d201" = 6.9
  dimension "d202" = 6.9
  dimension "d203" = 6.9
  text T0 "+" font "Arial" height 6.9 bold align left top in box 5.5016 x 4.0664 at (-31.9332, -38.7504) x (1, 0) y (0, 1) spacing 1 kerned
  text T1 "+" font "Arial" height 6.9 bold align left top in box 5.5016 x 4.0664 at (-24.9332, -38.7504) x (1, 0) y (0, 1) spacing 1 kerned
  text T2 "-" font "Arial" height 6.9 bold align left top in box 6.6976 x 2.392 at (-32.1724, -45.0892) x (1, 0) y (0, 1) spacing 1 kerned
  text T3 "-" font "Arial" height 6.9 bold align left top in box 6.6976 x 2.392 at (-22.1724, -45.0892) x (1, 0) y (0, 1) spacing 1 kerned
  text T4 "In" font "Arial" height 6.9 bold align left top in box 12.3188 x 6.578 at (-11.0032, -40.066) x (1, 0) y (0, 1) spacing 1 kerned
  text T5 "Out" font "Arial" height 6.9 bold align left top in box 13.6344 x 5.2624 at (-10.166, -47.9597) x (1, 0) y (0, 1) spacing 1 kerned
extrude "Lettering" add sketch "text Fills" along normal blind 1.5 separate body text T1 T0 T2 T3 T5 T4 makes body 3 at (-7.8603, -37.86, 0) makes body 4 at (3.9964, -47.0509, 0) makes body 5 at (-21.3064, -42.6972, 0.5) makes body 6 at (-27.7129, -37.3025, 0) makes body 7 at (-20.7129, -37.3025, 0) makes body 8 at (-31.3064, -42.6972, 0.5) makes body 9 at (1.6829, -47.0935, 0) makes body 10 at (-3.9863, -46.5773, 0) makes body 11 at (-11.0032, -38.088, 0.5)
move_body "Move6" bodies 2 to x (1, 0, 0) y (0, 1, 0) z (0, 0, 1) at (0, 0, 20) in component "Lid"
component "Lid" placed x (1, 0, 0) y (0, 1, 0) z (0, 0, 1) at (0, 0, 0)
named bodies: "Main box body", "Lid top", "+ (1)", "- (1)"
